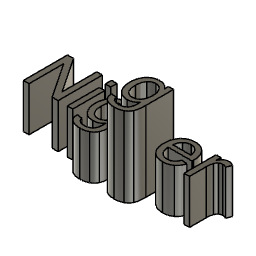
n v2 (Autodesk Fusion 360 design; units mm, degrees)
Autodesk Fusion 360 part; units mm, degrees
note: some values were not read from the file. Chosen so that the rebuilt part matches the saved one: which bodies a step acts on.
sketch "Sketch1" plane through (0, 0, 0) normal (0, 0, 1) x (1, 0, 0)
  line L0 (-86.7846, 1.4806) -> (23.0059, 1.4806) construction
  line L1 (23.0059, 1.4806) -> (23.0059, 36.5589) construction
  line L2 (23.0059, 36.5589) -> (-86.7846, 36.5589) construction
  line L3 (-86.7846, 36.5589) -> (-86.7846, 1.4806) construction
  dimension "d1" = 10
  text T0 "Nigger\n" font "Arial" height 10 align left top in box 109.7905 x 35.0783 at (-86.7846, 1.4806) x (1, 0) y (0, 1) spacing 1
extrude "Extrude1" add sketch "Sketch1" along normal blind 10 text T0 makes body 1 at (-76.8323, 35.6175, 3.3333) makes body 2 at (-50.4408, 28.9736, 3.3333) makes body 3 at (-60.052, 31.7158, 3.3333) makes body 4 at (-53.7355, 29.8672, 3.3333) makes body 5 at (-67.8214, 31.7158, 3.3333) makes body 6 at (-76.8323, 28.9736, 3.3333) makes body 7 at (-86.7846, 29.8922, 3.3333)
extrude "Extrude2" add 1 faces at (-60.434, 30.5379, 10) along direction (0, 0, 1) blind 8 on bodies 3 bodies 3
